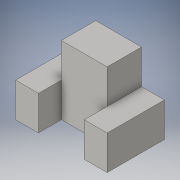
# Autodesk Inventor part: Figure 7_27_7
Saved by Autodesk Inventor 2016 (Build 200138000, 138)
## iProperties
Created: 2016-07-18
Part Number: Figure 7_27_7
Material: Generic
Document SubType Name: Modeling
Designer: cfkguest
Density: 1 g/cm^3
Appearance: Default
Author: cfkguest
Autodesk Inventor part; units mm, degrees
ref_plane "YZ Plane" through (0, 0, 0) normal (1, 0, 0) x (0, 1, 0)
ref_plane "XZ Plane" through (0, 0, 0) normal (0, 1, 0) x (-1, 0, 0)
ref_plane "XY Plane" through (0, 0, 0) normal (0, 0, 1) x (1, 0, 0)
sketch "Sketch1" plane through (0, 0, 0) normal (0, 0, 1) x (1, 0, 0)
  line L0 (-18.3251, 8.6116) -> (32.4749, 8.6116)
  line L1 (32.4749, 8.6116) -> (32.4749, -29.4884)
  line L2 (32.4749, -29.4884) -> (-18.3251, -29.4884)
  line L3 (-18.3251, -29.4884) -> (-18.3251, 8.6116)
  point P0 (0, 0)
  dimension "d0" = 50.8
  dimension "d1" = 38.1
  constraints: 8 end point, 2 parallel, 1 horizontal, 1 perpendicular
  measures "d0" distance of L0.start L0.end
  measures "d1" distance of L2.end L0.start
extrude "Extrusion1" add sketch "Sketch1" along normal blind 31.75
sketch "Sketch2" plane through (-18.3251, 8.6116, 0) normal (0, 1, 0) x (1, 0, 0)
  line L0 (50.8, -31.75) -> (0, -31.75) projected
  line L1 (12.7, -31.75) -> (38.1, -31.75)
  line L2 (38.1, -31.75) -> (38.1, -19.05)
  line L3 (38.1, -19.05) -> (12.7, -19.05)
  line L4 (12.7, -19.05) -> (12.7, -31.75)
  line L5 (50.8, 0) -> (50.8, -31.75) projected
  point P0 (18.3251, 0)
  dimension "d4" = 12.7
  dimension "d5" = 25.4
  dimension "d6" = 12.7
  constraints: 8 end point, 2 parallel, 1 horizontal, 1 perpendicular, 1 point on line
  measures "d4" distance of L3.end L1.start
  measures "d5" distance of L2.end L3.end
  measures "d6" distance between parallel lines of L5 L2
extrude "Extrusion2" cut sketch "Sketch2" against normal blind 38.1
sketch "Sketch3" plane through (0, 0, 31.75) normal (0, 0, 1) x (1, 0, 0)
  line L0 (32.4749, -29.4884) -> (32.4749, 8.6116) projected
  line L1 (19.7749, 8.6116) -> (32.4749, 8.6116)
  line L2 (32.4749, 8.6116) -> (32.4749, -10.4384)
  line L3 (32.4749, -10.4384) -> (19.7749, -10.4384)
  line L4 (19.7749, -10.4384) -> (19.7749, 8.6116)
  line L5 (-5.6251, 8.6116) -> (-18.3251, 8.6116) projected
  line L6 (-5.6251, -29.4884) -> (-5.6251, 8.6116) projected
  line L7 (-18.3251, 8.6116) -> (-5.6251, 8.6116)
  line L8 (-5.6251, 8.6116) -> (-5.6251, -10.4384)
  line L9 (-5.6251, -10.4384) -> (-18.3251, -10.4384)
  line L10 (-18.3251, -10.4384) -> (-18.3251, 8.6116)
  line L11 (-18.3251, -29.4884) -> (-5.6251, -29.4884) projected
  line L12 (19.7749, -29.4884) -> (32.4749, -29.4884) projected
  point P0 (0, 0)
  dimension "d9" = 19.05
  dimension "d10" = 19.05
  constraints: 16 end point, 4 parallel, 2 horizontal, 2 midpoint, 2 perpendicular
  measures "d9" distance between parallel lines of L11 L9
  measures "d10" distance between parallel lines of L12 L3
extrude "Extrusion3" cut sketch "Sketch3" against normal blind 38.1
body "Solid1"
